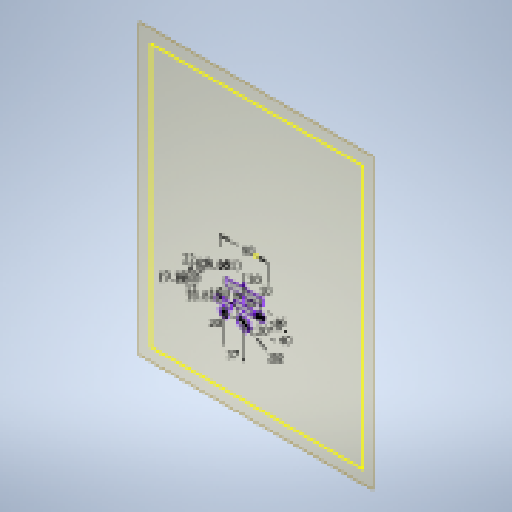
# Autodesk Inventor part: mode-control-layout
Saved by Autodesk Inventor 2023 (Build 270158030, 158C)
## iProperties
Created: 2024-04-02
Part Number: mode-control-layout
Material: Generic
Document SubType Name: Modeling
Designer: Imogen Heard
Density: 1 g/cm^3
Appearance: Default
Author: Imogen Heard
Autodesk Inventor part; units mm, degrees
ref_plane "YZ Plane" through (0, 0, 0) normal (1, 0, 0) x (0, 1, 0)
ref_plane "XZ Plane" through (0, 0, 0) normal (0, 1, 0) x (-1, 0, 0)
ref_plane "XY Plane" through (0, 0, 0) normal (0, 0, 1) x (1, 0, 0)
ref_plane "Work Plane1" through (0, 0, 0) normal (0, 0, 1) x (1, 0, 0)
sketch "Sketch1" plane through (0, 0, 0) normal (0, 0, 1) x (1, 0, 0)
  line L0 (-68.1954, -80.0527) -> (21.8046, -80.0527) construction
  line L1 (21.8046, -80.0527) -> (21.8046, -58.0527) construction
  line L2 (21.8046, -58.0527) -> (-68.1954, -58.0527) construction
  line L3 (-68.1954, -58.0527) -> (-68.1954, -80.0527) construction
  circle A0 centre (-23.1954, -120.0527) radius 11
  line L4 (-40.6954, -100.0527) -> (-5.6954, -100.0527) construction
  line L5 (-5.6954, -100.0527) -> (-5.6954, -90.0527) construction
  line L6 (-5.6954, -90.0527) -> (-40.6954, -90.0527) construction
  line L7 (-40.6954, -90.0527) -> (-40.6954, -100.0527) construction
  line L8 (-75.1954, -99.2393) -> (-75.1954, -109.2393) construction
  line L9 (-75.1954, -109.2393) -> (-45.1954, -109.2393) construction
  line L10 (-45.1954, -109.2393) -> (-45.1954, -99.2393) construction
  line L11 (-45.1954, -99.2393) -> (-75.1954, -99.2393) construction
  circle A1 centre (-23.1954, -120.0527) radius 14.5 construction
  circle A2 centre (6.8046, -95.0527) radius 8
  circle A3 centre (-60.1954, -121.2393) radius 8
  circle A4 centre (6.8046, -95.0527) radius 10 construction
  circle A5 centre (-60.1954, -121.2393) radius 10 construction
  line L12 (-198, -244.5) -> (198, -244.5) projected
  line L13 (198, -244.5) -> (198, 244.5) projected
  line L14 (198, 244.5) -> (-198, 244.5) projected
  line L15 (-198, 244.5) -> (-198, -244.5) projected
  line L16 (-75.1954, -99.2393) -> (-45.1954, -99.2393)
  line L17 (-45.1954, -99.2393) -> (-45.1954, -109.2393)
  line L18 (-45.1954, -109.2393) -> (-75.1954, -109.2393)
  line L19 (-75.1954, -109.2393) -> (-75.1954, -99.2393)
  line L20 (-40.6954, -90.0527) -> (-5.6954, -90.0527)
  line L21 (-5.6954, -90.0527) -> (-5.6954, -100.0527)
  line L22 (-5.6954, -100.0527) -> (-40.6954, -100.0527)
  line L23 (-40.6954, -100.0527) -> (-40.6954, -90.0527)
  line L24 (-58.1954, -62.8527) -> (11.8046, -62.8527)
  line L25 (11.8046, -62.8527) -> (11.8046, -75.7527)
  line L26 (11.8046, -75.7527) -> (-58.1954, -75.7527)
  line L27 (-58.1954, -75.7527) -> (-58.1954, -62.8527)
  point P0 (0, 0)
  point P1 (-23.1954, -80.0527)
  point P2 (-23.1954, -100.0527)
  point P3 (-60.1954, -99.2393)
  point P4 (-60.1954, -109.2393)
  point P5 (-5.6954, -95.0527)
  point P6 (-23.1954, -90.0527)
  point P7 (-23.1954, -58.0527)
  dimension "d0" = 22
  dimension "d1" = 22
  dimension "d2" = 90
  dimension "d7" = 29
  dimension "d8" = 16
  dimension "d9" = 16
  dimension "d10" = 20
  dimension "d11" = 20
  dimension "d12" = 30
  dimension "d14" = 40
  dimension "d17" = 37
  dimension "d18" = 20
  dimension "d19" = 10
  dimension "d20" = 10
  dimension "d21" = 30
  dimension "d22" = 35
  dimension "d26" = 39.0513
  dimension "d28" = 4.3
  dimension "d29" = 4.8
  dimension "d30" = 10
  dimension "d31" = 10
  dimension "d124" = 10.8134
  dimension "d125" = 9.1866
  dimension "d126" = 12
  constraints: 24 end point, 7 midpoint, 6 centre point, 6 parallel, 6 vertical alignment, 4 coincident, 3 horizontal, 3 perpendicular, 1 horizontal alignment, 6 other
  measures "d0" diameter of A0
  measures "d1" distance between parallel lines of L0 L2
  measures "d2" distance between parallel lines of L1 L3
  measures "d7" diameter of A1
  measures "d8" diameter of A2
  measures "d9" diameter of A3
  measures "d10" diameter of A4
  measures "d11" diameter of A5
  measures "d12" horizontal distance of A2.centre point (-23.195, -100.053)
  measures "d14" distance from line of A0.centre L0
  measures "d17" horizontal distance of A3.centre A0.centre
  measures "d18" distance from line of A0.centre L4
  measures "d19" distance between parallel lines of L4 L6
  measures "d20" distance between parallel lines of L9 L11
  measures "d21" distance between parallel lines of L10 L8
  measures "d22" distance between parallel lines of L5 L7
  measures "d26" distance of A0.centre A4.centre
  measures "d28" distance between parallel lines of L0 L26
  measures "d29" distance between parallel lines of L2 L24
  measures "d30" distance between parallel lines of L1 L25
  measures "d31" distance between parallel lines of L3 L27
  measures "d124" distance from line of L9 A0.centre
  measures "d125" distance between parallel lines of L4 L9
  measures "d126" distance from line of L18 A3.centre
extrude "Extrusion1" add sketch "Sketch1" along normal blind 1 contours A0 | A2 | A3 | L16 L17 L18 L19 | L20 L21 L22 L23 | L24 L25 L26 L27
sketch "Sketch5" plane through (0, 0, 1) normal (0, 0, 1) x (1, 0, 0)
  line L0 (-55.571, -65.5595) -> (9.6532, -65.5595) construction
  line L1 (9.6532, -65.5595) -> (9.6532, -73.7983) construction
  line L2 (9.6532, -73.7983) -> (-55.571, -73.7983) construction
  line L3 (-55.571, -73.7983) -> (-55.571, -65.5595) construction
  point P0 (0, 0)
  constraints: 1 horizontal, 2 other
decal "Decal1"
sketch "Sketch6" plane through (0, 0, 1) normal (0, 0, 1) x (1, 0, 0)
  line L0 (-73.1954, -100.8393) -> (-47.3362, -100.8393) construction
  line L1 (-47.3362, -100.8393) -> (-47.3362, -107.6393) construction
  line L2 (-47.3362, -107.6393) -> (-73.1954, -107.6393) construction
  line L3 (-73.1954, -107.6393) -> (-73.1954, -100.8393) construction
  line L4 (-75.1954, -109.2393) -> (-45.1954, -109.2393) projected
  line L5 (-45.1954, -99.2393) -> (-75.1954, -99.2393) projected
  line L6 (-75.1954, -99.2393) -> (-75.1954, -109.2393) projected
  point P0 (0, 0)
  point P1 (-75.1954, -104.2393)
  dimension "d130" = 1.6
  dimension "d131" = 1.6
  dimension "d132" = 2
  constraints: 1 horizontal, 1 midpoint, 2 other
  measures "d130" distance between parallel lines of L4 L2
  measures "d131" distance between parallel lines of L5 L0
  measures "d132" distance from line of point (-75.195, -104.239) L3
decal "Decal2"
sketch "Sketch7" plane through (0, 0, 1) normal (0, 0, 1) x (1, 0, 0)
  line L0 (-38.5335, -91.962) -> (-7.4329, -91.962) construction
  line L1 (-7.4329, -91.962) -> (-7.4329, -98.548) construction
  line L2 (-7.4329, -98.548) -> (-38.5335, -98.548) construction
  line L3 (-38.5335, -98.548) -> (-38.5335, -91.962) construction
  point P0 (0, 0)
  constraints: 2 other
decal "Decal3"
